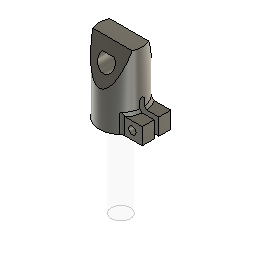
Holder for 8mm Shaft (Autodesk Fusion 360 design; units mm, degrees)
Autodesk Fusion 360 part; units mm, degrees
cylinder "CylinderPrimitive1" add diameter 8 height 50 placed x (1, 0, 0) y (0, 1, 0) z (0, 0, 1) at (0, 0, 0) makes body 1 in component "8mm rod"
sketch "Sketch1" plane through (0, 0, 50) normal (0, 0, 1) x (-1, 0, 0) in component "8mmRodHolder"
  circle A0 centre (0, 0) radius 4
  circle A1 centre (0, 0) radius 9
  dimension "d4" = 5
  constraint concentric A0 A1
  measures "d4" distance of A0 A1
extrude "Extrude1" add sketch "Sketch1" against normal blind 15 separate body makes body 2 in component "8mmRodHolder"
extrude "Extrude2" add sketch "Sketch1" along normal blind 15 contours A0 | A1 bodies 2 in component "8mmRodHolder"
ref_plane "WorkPlane1" through (9, 0, 59.0241) normal (1, 0, 0) x (0, 1, 0) in component "8mmRodHolder"
sketch "Sketch2" plane through (9, 0, 0) normal (1, 0, 0) x (0, 1, 0) in component "8mmRodHolder"
  line L0 (9, 65) -> (-9, 65)
  line L1 (-9, 35) -> (9, 35)
  line L2 (9, 50) -> (-9, 50)
  line L3 (9, 50) -> (3.5, 65)
  line L4 (0, 50) -> (0, 58)
  line L5 (-9, 50) -> (-3.5, 65)
  line L6 (9, 65) -> (9, 50)
  line L7 (-9, 65) -> (-9, 50)
  line L8 (1, 35) -> (1, 47)
  line L9 (-1, 35) -> (-1, 47)
  line L10 (1, 47) -> (-1, 47)
  line L11 (6, 35) -> (6, 42)
  line L12 (-6, 35) -> (-6, 42)
  line L13 (6, 42) -> (1, 42)
  line L14 (-1, 42) -> (-6, 42)
  line L15 (1, 42) -> (-1, 42) construction
  dimension "d10" = 7
  dimension "d11" = 2
  dimension "d12" = 3
  dimension "d14" = 8
  dimension "d16" = 5
  dimension "d17" = 7
  constraint coincident L2.start L3.start
  constraint coincident L0 L3.end
  constraint midpoint L2 L4.start
  constraint perpendicular L2 L4
  constraint symmetric L2.start L4 L2.end
  constraint symmetric L3.end L4 L5.end
  constraint coincident L0.start L6.start
  constraint coincident L0.end L7.start
  constraint coincident L2.end L5.start
  constraint coincident L1 L8.start
  constraint perpendicular L1 L8
  constraint symmetric L4 L8.start L9.start
  constraint symmetric L4 L8.end L9.end
  constraint coincident L1 L11.start
  constraint perpendicular L1 L11
  constraint symmetric L4 L11.start L12.start
  constraint symmetric L4 L11.end L12.end
  constraint coincident L12.end L14.end
  constraint coincident L8 L13.end
  constraint coincident L9 L14.start
  constraint collinear L13 L14
  measures "d10" distance of L3.end L5.end
  measures "d11" distance of L8.end L9.end
  measures "d12" distance of L2 L10
  measures "d14" distance of L4.start L4.end
  measures "d16" distance of L11.end L13.end
  measures "d17" distance of L11.start L11.end
extrude "Extrude3" add sketch "Sketch2" along normal blind 6 and the other way up to surface contours L1 L9 L12 L14 | L1 L8 L11 L13 second end surface at (-8.9553, 0.8961, 45) on bodies 2 bodies 2 in component "8mmRodHolder"
extrude "Extrude4" cut sketch "Sketch2" against normal through all contours L0 L3 L6 | L0 L5 L7 bodies 2 in component "8mmRodHolder"
extrude "Extrude5" cut sketch "Sketch2" against normal blind 9 contours L1 L8 L9 L10 bodies 2 in component "8mmRodHolder"
sketch "Sketch3" plane through (0, 6, 0) normal (0, 1, 0) x (-1, 0, 0) in component "8mmRodHolder"
  line L0 (-6.7082, 42) -> (-15, 42)
  line L1 (-15, 42) -> (-15, 35)
  line L2 (-15, 35) -> (-6.7082, 35)
  line L3 (-6.7082, 35) -> (-6.7082, 42)
  line L4 (-8.9443, 47) -> (-8.9443, 42)
  line L5 (-8.2916, 65) -> (8.2916, 65)
  ellipse E0 centre (0, 74.5455) end of major axis (0, 50) minor radius 9 (-8.2916, 65) -> (8.2916, 65) ccw
  line L6 (-15, 35) -> (-15, 42)
  line L7 (0, 65) -> (0, 58) construction
  line L8 (2.4749, 60.4749) -> (5.2341, 57.7157) construction
  line L9 (2.4749, 60.4749) -> (-2.4749, 60.4749)
  arc A0 (-2.4749, 60.4749) -> (2.4749, 60.4749) centre (0, 58) ccw
  arc A1 (0, 61.5) -> (-2.4749, 60.4749) centre (0, 58) ccw construction
  arc A2 (2.4749, 60.4749) -> (0, 61.5) centre (0, 58) ccw construction
  line L10 (-15, 42) -> (-6.7082, 35) construction
  circle A3 centre (-10.8541, 38.5) radius 1.55
  dimension "d25" = 7
  dimension "d26" = 7
  dimension "d27" = 45
  dimension "d28" = 3.1
  constraint midpoint L5 L7.start
  constraint perpendicular L5 L7
  constraint coincident L7.end A0.centre
  constraint tangent L8 A0
  constraint perpendicular L7 L9
  constraint coincident L7 A1.start
  constraint concentric A0 A1
  constraint concentric A0 A2
  constraint coincident L0.end L1.start
  constraint coincident L2.end L3.start
  constraint midpoint L10 A3.centre
  measures "d25" distance of L7.start L7.end
  measures "d26" diameter of A0
  measures "d27" angle of L7 L8
  measures "d28" diameter of A3
extrude "Extrude6" cut sketch "Sketch3" against normal through all and the other way through all contours L9 A0 | A3 bodies 2 in component "8mmRodHolder"
fillet "Fillet1" radius 2 2 edges at (6.7082, -6, 38.5) (6.7082, 6, 38.5) on bodies 2 in component "8mmRodHolder"
chamfer "Chamfer1" distance 1 angle 45 2 edges at (8.0531, -4.0184, 42) (8.0531, 4.0184, 42) on bodies 2 in component "8mmRodHolder"
chamfer "Chamfer2" distance 1 angle 45 2 edges at (6.4086, -1, 47) (6.4086, 1, 47) on bodies 2 in component "8mmRodHolder"
component "8mm rod" placed x (1, 0, 0) y (0, 1, 0) z (0, 0, 1) at (0, 0, 0)
component "8mmRodHolder" placed x (1, 0, 0) y (0, 1, 0) z (0, 0, 1) at (0, 0, 0)
named bodies: "Sample8mmRod", "8mmRodHolder"
